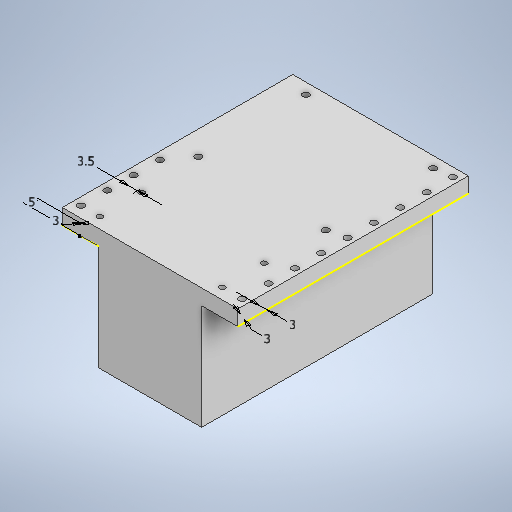
# Autodesk Inventor part: battery_holder
Saved by Autodesk Inventor 2025 (Build 290162010, 162A)
## iProperties
Created: 2024-10-24
Part Number: battery_holder
Material: Generic
Document SubType Name: Modeling
Designer: fist5
Density: 1 g/cm^3
Appearance: Default
Author: fist5
Autodesk Inventor part; units mm, degrees
ref_plane "YZ Plane" through (0, 0, 0) normal (1, 0, 0) x (0, 1, 0)
ref_plane "XZ Plane" through (0, 0, 0) normal (0, 1, 0) x (-1, 0, 0)
ref_plane "XY Plane" through (0, 0, 0) normal (0, 0, 1) x (1, 0, 0)
sketch "Sketch3" plane through (0, 0, 0) normal (0, 1, 0) x (-1, 0, 0)
  line L0 (47, 105) -> (0, 105)
  line L1 (0, 105) -> (0, 0)
  line L2 (0, 0) -> (47, 0)
  line L3 (47, 0) -> (47, 105)
  line L4 (37, 95) -> (10, 95)
  line L5 (10, 95) -> (10, 0)
  line L6 (10, 0) -> (37, 0)
  line L7 (37, 0) -> (37, 95)
  point P0 (37, 0)
  dimension "d8" = 10
  dimension "d9" = 10
  dimension "d10" = 10
  dimension "d11" = 27
  dimension "d12" = 95
  constraints: 16 end point, 4 parallel, 2 horizontal, 2 perpendicular, 1 coincident, 1 point on line
  measures "d8" distance between parallel lines of L0 L4
  measures "d9" distance between parallel lines of L1 L5
  measures "d10" distance between parallel lines of L3 L7
  measures "d11" distance between parallel lines of L5 L7
  measures "d12" distance between parallel lines of L4 L2
extrude "Extrusion1" add sketch "Sketch3" along normal blind 45 contours L3 L2 L7 L4 L5 L1 L0
sketch "Sketch4" plane through (0, 45, 0) normal (0, 1, 0) x (1, 0, 0)
  line L0 (-47, 0) -> (-47, -105) projected
  line L1 (0, -105) -> (0, 0) projected
  line L2 (-47, -105) -> (0, -105)
  line L3 (0, -105) -> (0, 0)
  line L4 (0, 0) -> (-47, 0)
  line L5 (-47, 0) -> (-47, -105)
  point P0 (0, -105)
  constraints: 8 end point, 2 parallel, 1 horizontal, 1 perpendicular
extrude "Extrusion2" add sketch "Sketch4" along normal blind 10
sketch "Sketch5" plane through (0, 55, 0) normal (0, 1, 0) x (1, 0, 0)
  line L0 (0, 0) -> (-10, 0) projected
  line L1 (0, 0) -> (16.5, 0)
  line L2 (16.5, 0) -> (16.5, -105)
  line L3 (16.5, -105) -> (0, -105)
  line L4 (0, -105) -> (0, 0)
  line L5 (-47, 0) -> (-47, -105) projected
  line L6 (-47, 0) -> (-63.5, 0)
  line L7 (-63.5, 0) -> (-63.5, -105)
  line L8 (-63.5, -105) -> (-47, -105)
  line L9 (-47, -105) -> (-47, 0)
  line L10 (0, 0) -> (-47, 0) projected
  point P0 (-23.5, 0)
  dimension "d17" = 40
  dimension "d18" = 80
  constraints: 16 end point, 4 parallel, 2 horizontal, 2 horizontal alignment, 2 perpendicular, 1 midpoint
  measures "d17" distance from line of point (-23.5, 0) L7
  measures "d18" distance between parallel lines of L7 L2
extrude "Extrusion3" add sketch "Sketch5" against normal blind 7
sketch "Sketch7" plane through (0, 0, 0) normal (0, -1, 0) x (1, 0, 0)
  line L0 (-42, 0) -> (-5, 0)
  line L1 (-5, 0) -> (-5, 100)
  line L2 (-5, 100) -> (-42, 100)
  line L3 (-42, 100) -> (-42, 0)
  line L4 (-47, 0) -> (-47, 105) projected
  line L5 (0, 105) -> (0, 0) projected
  line L6 (-47, 105) -> (0, 105) projected
  circle A0 centre (-42, 100) radius 1.5
  dimension "d21" = 5
  dimension "d22" = 5
  dimension "d23" = 5
  dimension "d24" = 3
  constraints: 8 end point, 2 parallel, 1 centre point, 1 coincident, 1 horizontal, 1 horizontal alignment, 1 perpendicular
  measures "d21" distance between parallel lines of L4 L3
  measures "d22" distance between parallel lines of L5 L1
  measures "d23" distance between parallel lines of L6 L2
  measures "d24" diameter of A0
extrude "Extrusion4" cut sketch "Sketch7" against normal blind 10 contours A0 L2 L3 | L3 L2 A0
sketch "Sketch8" plane through (0, 0, 0) normal (0, -1, 0) x (1, 0, 0)
  circle A0 centre (-42, 100) radius 1.5 projected
  line L0 (-42, 103.1754) -> (-39.25, 101.5877)
  line L1 (-39.25, 101.5877) -> (-39.25, 98.4123)
  line L2 (-39.25, 98.4123) -> (-42, 96.8246)
  line L3 (-42, 96.8246) -> (-44.75, 98.4123)
  line L4 (-44.75, 98.4123) -> (-44.75, 101.5877)
  line L5 (-44.75, 101.5877) -> (-42, 103.1754)
  line L6 (-47, 0) -> (-47, 105) projected
  point P0 (0, 0)
  point P1 (-39.25, 100)
  dimension "d27" = 5.5
  constraints: 12 end point, 1 coincident, 1 midpoint, 1 parallel, 13 other
  measures "d27" distance from line of point (-39.25, 100) L4
extrude "Extrusion5" cut sketch "Sketch8" against normal blind 3.3
pattern_linear "Rectangular Pattern1" count 5 spacing 23 along (0, 0, -1) count 2 spacing 37 along (1, 0, 0) of "Extrusion4", "Extrusion5"
sketch "Sketch9" plane through (-47, 0, 0) normal (-1, 0, 0) x (0, 0, 1)
  line L0 (36, 40.5) -> (95, 40.5)
  line L1 (95, 40.5) -> (95, 7.5)
  line L2 (95, 7.5) -> (36, 7.5)
  line L3 (36, 7.5) -> (36, 40.5)
  line L4 (98.5, 3.3) -> (101.5, 3.3) projected
  line L5 (101.5, 10) -> (98.5, 10) projected
  line L6 (0, 0) -> (105, 0) projected
  line L7 (105, 0) -> (105, 48) projected
  circle A0 centre (36, 40.5) radius 1.5
  circle A1 centre (95, 40.5) radius 1.5
  circle A2 centre (95, 7.5) radius 1.5
  circle A3 centre (36, 7.5) radius 1.5
  point P0 (95, 24)
  dimension "d36" = 33
  dimension "d38" = 24
  dimension "d39" = 10
  dimension "d40" = 59
  dimension "d41" = 3
  dimension "d42" = 3
  dimension "d43" = 3
  dimension "d44" = 3
  constraints: 8 end point, 4 centre point, 4 coincident, 2 parallel, 1 horizontal, 1 midpoint, 1 perpendicular
  measures "d36" distance between parallel lines of L2 L0
  measures "d38" distance from line of L6 point (95, 24)
  measures "d39" distance between parallel lines of L7 L1
  measures "d40" distance between parallel lines of L1 L3
  measures "d41" diameter of A0
  measures "d42" diameter of A3
  measures "d43" diameter of A1
  measures "d44" diameter of A2
extrude "Extrusion6" cut sketch "Sketch9" against normal blind 5 contours L3 A0 L0 | L0 A0 L3 | A1 L1 L0 | L0 L1 A1 | A3 L2 L3 | L3 L2 A3 | A2 L2 L1 | L1 L2 A2
sketch "Sketch10" plane through (-47, 0, 0) normal (-1, 0, 0) x (0, 0, 1)
  line L0 (5, 34.25) -> (22.25, 34.25)
  line L1 (22.25, 34.25) -> (22.25, 13.75)
  line L2 (22.25, 13.75) -> (5, 13.75)
  line L3 (5, 13.75) -> (5, 34.25)
  line L4 (0, 0) -> (105, 0) projected
  line L5 (0, 0) -> (0, 48) projected
  circle A0 centre (5, 34.25) radius 1.25
  circle A1 centre (22.25, 34.25) radius 1.25
  circle A2 centre (5, 13.75) radius 1.25
  circle A3 centre (22.25, 13.75) radius 1.25
  point P0 (5, 24)
  point P1 (0, 24)
  dimension "d47" = 17.25
  dimension "d48" = 20.5
  dimension "d49" = 24
  dimension "d50" = 5
  dimension "d51" = 2.5
  dimension "d52" = 2.5
  dimension "d53" = 2.5
  dimension "d54" = 2.5
  constraints: 8 end point, 4 centre point, 4 coincident, 2 midpoint, 2 parallel, 1 horizontal, 1 perpendicular
  measures "d47" distance between parallel lines of L1 L3
  measures "d48" distance between parallel lines of L2 L0
  measures "d49" distance from line of L4 point (5, 24)
  measures "d50" distance of point (0, 24) point (5, 24)
  measures "d51" diameter of A1
  measures "d52" diameter of A3
  measures "d53" diameter of A0
  measures "d54" diameter of A2
extrude "Extrusion7" cut sketch "Sketch10" against normal blind 5 contours L3 A0 L0 | L0 A0 L3 | A1 L1 L0 | L0 L1 A1 | A2 L2 L3 | L3 L2 A2 | A3 L2 L1 | L1 L2 A3
sketch "Sketch11" plane through (0, 55, 0) normal (0, 1, 0) x (1, 0, 0)
  line L0 (-51.44, -100) -> (4.44, -100)
  line L1 (4.44, -100) -> (4.44, -80.95)
  line L2 (4.44, -80.95) -> (-51.44, -80.95)
  line L3 (-51.44, -80.95) -> (-51.44, -100)
  line L4 (-52.5, -54) -> (5.5, -54)
  line L5 (5.5, -54) -> (5.5, -5)
  line L6 (5.5, -5) -> (-52.5, -5)
  line L7 (-52.5, -5) -> (-52.5, -54)
  line L8 (16.5, -105) -> (16.5, 0) projected
  line L9 (16.5, 0) -> (-63.5, 0) projected
  line L10 (-63.5, -105) -> (16.5, -105) projected
  circle A0 centre (-51.44, -100) radius 1.25
  circle A1 centre (-51.44, -80.95) radius 1.25
  circle A2 centre (4.44, -100) radius 1.25
  circle A3 centre (4.44, -80.95) radius 1.25
  circle A4 centre (-52.5, -54) radius 1.5
  line L11 (5.5, 44) -> (-52.5, 44)
  circle A5 centre (-52.5, -5) radius 1.5
  line L12 (63.5, -5) -> (5.5, -5)
  circle A6 centre (5.5, -54) radius 1.5
  line L13 (63.5, 44) -> (5.5, 44)
  circle A7 centre (5.5, -5) radius 1.5
  point P0 (0, 0)
  point P1 (-23.5, -5)
  point P2 (-23.5, -100)
  point P3 (-23.5, 44)
  point P4 (34.5, -5)
  point P5 (34.5, 44)
  dimension "d57" = 58
  dimension "d58" = 40
  dimension "d59" = 49
  dimension "d60" = 5
  dimension "d61" = 5
  dimension "d62" = 19.05
  dimension "d63" = 55.88
  dimension "d64" = 40
  dimension "d65" = 2.5
  dimension "d68" = 19.05
  dimension "d71" = 55.88
  dimension "d74" = 3
  dimension "d77" = 49
  dimension "d80" = 58
  constraints: 22 end point, 8 centre point, 4 horizontal, 4 parallel, 2 coincident, 2 midpoint, 2 perpendicular, 2 vertical, 24 other
  measures "d57" distance between parallel lines of L5 L7
  measures "d58" distance from line of L8 point (-23.5, -5)
  measures "d59" distance between parallel lines of L4 L6
  measures "d60" distance between parallel lines of L9 L6
  measures "d61" distance from line of L10 point (-23.5, -100)
  measures "d62" distance between parallel lines of L0 L2
  measures "d63" distance between parallel lines of L1 L3
  measures "d64" distance from line of L8 point (-23.5, -100)
  measures "d65" diameter of A0
  measures "d68" distance of A0.centre A1.centre
  measures "d71" distance of A0.centre A2.centre
  measures "d74" diameter of A4
  measures "d77" distance of L5.end L11.start
  measures "d80" distance of L5.end L12.start
extrude "Extrusion8" cut sketch "Sketch11" against normal up to next contours L3 A0 L0 | L0 A0 L3 | A2 L1 L0 | L0 L1 A2 | A1 L2 L3 | L3 L2 A1 | A3 L2 L1 | L1 L2 A3 | L7 A4 L4 | L4 A4 L7 | A6 L5 L4 | L4 L5 A6 | A5 L6 L7 | L7 L6 A5 | A7 L6 L5 | L5 L12 A7 | A7 L12 L6
sketch "Sketch12" plane through (0, 48, 0) normal (0, -1, 0) x (1, 0, 0)
  line L0 (-60, 100) -> (13.5, 100)
  line L1 (13.5, 100) -> (13.5, 0)
  line L2 (13.5, 0) -> (-60, 0)
  line L3 (-60, 0) -> (-60, 100)
  line L4 (-47, 105) -> (-63.5, 105) projected
  line L5 (-63.5, 105) -> (-63.5, 0) projected
  line L6 (16.5, 0) -> (16.5, 105) projected
  circle A0 centre (-60, 100) radius 1.5
  circle A1 centre (13.5, 100) radius 1.5
  point P0 (0, 0)
  point P1 (-55.25, 105)
  dimension "d85" = 5
  dimension "d86" = 3.5
  dimension "d87" = 3
  dimension "d88" = 3
  dimension "d89" = 3
  constraints: 8 end point, 2 centre point, 2 coincident, 2 parallel, 1 horizontal, 1 horizontal alignment, 1 midpoint, 1 perpendicular
  measures "d85" distance from line of point (-55.25, 105) L0
  measures "d86" distance between parallel lines of L5 L3
  measures "d87" distance between parallel lines of L6 L1
  measures "d88" diameter of A0
  measures "d89" diameter of A1
extrude "Extrusion9" cut sketch "Sketch12" against normal up to next contours L3 A0 L0 | L0 A0 L3
pattern_linear "Rectangular Pattern2" count 4 spacing 12 along (0, 0, -1) of "Extrusion9"
extrude "Extrusion10" cut sketch "Sketch12" against normal up to next contours A1 L1 L0 | L0 L1 A1
pattern_linear "Rectangular Pattern3" count 9 spacing 12 along (0, 0, -1) of "Extrusion10"
body "Solid1"
